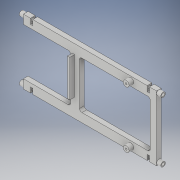
# Autodesk Inventor part: Drivercarrier
Saved by Autodesk Inventor 2019 (Build 230136000, 136)
## iProperties
Created: 2019-01-03
Part Number: Drivercarrier
Material: Generic
Document SubType Name: Modeling
Designer: Martin
Density: 1 g/cm^3
Appearance: Default
Author: Martin
Autodesk Inventor part; units mm, degrees
ref_plane "YZ Plane" through (0, 0, 0) normal (1, 0, 0) x (0, 1, 0)
sketch "Sketch1" plane through (0, 0, 0) normal (0, 0, 1) x (1, 0, 0)
  line L0 (-60, -27.5) -> (60, -27.5)
  line L1 (60, -27.5) -> (60, 27.5)
  line L2 (60, 27.5) -> (-60, 27.5)
  line L3 (-60, 27.5) -> (-60, -27.5)
  line L4 (-60, -27.5) -> (60, 27.5) construction
  line L5 (60, -27.5) -> (-60, 27.5) construction
  point P0 (0, 0)
  dimension "d0" = 120
  dimension "d1" = 55
  constraints: 12 end point, 2 midpoint, 2 parallel, 1 horizontal, 1 perpendicular
  measures "d0" distance of L2.end L1.end
  measures "d1" distance of L1.end L0.end
extrude "Extrusion1" add sketch "Sketch1" against normal blind 4
sketch "Sketch2" plane through (60, -27.5, 0) normal (1, 0, 0) x (0, 0, -1)
  circle A0 centre (2, 2) radius 2
  line L0 (0, 0) -> (4, 0) projected
  line L1 (4, 55) -> (4, 0) projected
  circle A1 centre (2, 2) radius 1.25
  circle A2 centre (2, 53) radius 2
  line L2 (0, 55) -> (4, 55) projected
  circle A3 centre (2, 53) radius 1.25
  line L3 (0, 55) -> (0, 0) projected
  line L4 (0, 55) -> (4, 55)
  line L5 (4, 55) -> (4, 0)
  line L6 (4, 0) -> (0, 0)
  line L7 (0, 0) -> (0, 55)
  point P0 (0, 27.5)
  dimension "d4" = 4
  dimension "d5" = 2.5
  dimension "d6" = 4
  dimension "d7" = 2.5
  constraints: 8 end point, 4 centre point, 4 tangent, 2 coincident, 2 parallel, 1 horizontal, 1 perpendicular
  measures "d4" diameter of A0
  measures "d5" diameter of A1
  measures "d6" diameter of A2
  measures "d7" diameter of A3
extrude "Extrusion2" cut sketch "Sketch2" against normal blind 3.5 contours L1 L0 A0 | A0 L3 A2 L1 | A0 L0 L3 | A2 L2 L1 | L3 L2 A2
extrude "Extrusion3" cut sketch "Sketch2" against normal blind 25 contours A1
extrude "Extrusion4" cut sketch "Sketch2" against normal blind 25 contours A3
sketch "Sketch3" plane through (-60, -27.5, 0) normal (-1, 0, 0) x (0, 0, 1)
  circle A0 centre (-2, 2) radius 2
  circle A1 centre (-2, 53) radius 2
  line L0 (0, 0) -> (-4, 0) projected
  line L1 (-4, 0) -> (-4, 55) projected
  line L2 (0, 55) -> (-4, 55) projected
  line L3 (0, 55) -> (0, 0) projected
  line L4 (-4, 0) -> (0, 0)
  line L5 (0, 0) -> (0, 55)
  line L6 (0, 55) -> (-4, 55)
  line L7 (-4, 55) -> (-4, 0)
  circle A2 centre (-2, 2) radius 1.25 projected
  circle A3 centre (-2, 2) radius 1.25
  circle A4 centre (-2, 53) radius 1.25 projected
  circle A5 centre (-2, 53) radius 1.25
  point P0 (0, 27.5)
  dimension "d14" = 4
  dimension "d15" = 4
  dimension "d16" = 2.5
  dimension "d17" = 2.5
  constraints: 8 end point, 4 centre point, 4 tangent, 2 coincident, 2 parallel, 1 horizontal, 1 perpendicular
  measures "d14" diameter of A0
  measures "d15" diameter of A1
  measures "d16" diameter of A3
  measures "d17" diameter of A5
extrude "Extrusion5" cut sketch "Sketch3" against normal blind 3.5 contours L3 L0 A0 | A0 L1 A1 L3 | A0 L0 L1 | A1 L2 L3 | L1 L2 A1
extrude "Extrusion6" cut sketch "Sketch3" against normal blind 25 contours A4
extrude "Extrusion7" cut sketch "Sketch3" against normal blind 25 contours A2
sketch "Sketch4" plane through (0, 0, 0) normal (0, 0, 1) x (1, 0, 0)
  line L0 (-56.5, 27.5) -> (56.5, 27.5) projected
  line L1 (56.5, -27.5) -> (-56.5, -27.5) projected
  line L2 (-56.5, 27.5) -> (56.5, 27.5)
  line L3 (56.5, 27.5) -> (56.5, -27.5)
  line L4 (56.5, -27.5) -> (-56.5, -27.5)
  line L5 (-56.5, -27.5) -> (-56.5, 27.5)
  line L6 (-73.441, 25.5) -> (75.6749, 25.5) construction
  line L7 (-49.5, 37.9771) -> (-49.5, -42.6684) construction
  line L8 (-50.45, 28) -> (-48.55, 28)
  line L9 (-48.55, 28) -> (-48.55, 23)
  line L10 (-48.55, 23) -> (-50.45, 23)
  line L11 (-50.45, 23) -> (-50.45, 28)
  line L12 (-50.45, 28) -> (-48.55, 23) construction
  line L13 (-48.55, 28) -> (-50.45, 23) construction
  point P0 (0, 0)
  point P1 (-49.5, 25.5)
  dimension "d24" = 2
  dimension "d25" = 7
  dimension "d26" = 1.9
  dimension "d27" = 5
  constraints: 24 end point, 4 parallel, 3 horizontal, 2 midpoint, 2 perpendicular, 2 point on line, 1 vertical
  measures "d24" distance between parallel lines of L0 L6
  measures "d25" distance between parallel lines of L7 L5
  measures "d26" distance of L9.end L10.end
  measures "d27" distance between parallel lines of L10 L8
extrude "Extrusion8" cut sketch "Sketch4" against normal blind 25 contours L11 L8 L9 L0 | L0 L9 L10 L11
ref_plane "Work Plane1" through (0, -27.5, 0) normal (1, 0, 0) x (0, 0, -1)
ref_plane "Work Plane2" through (-48.55, 0, 0) normal (0, 1, 0) x (1, 0, 0)
mirror "Mirror1" about plane through (0, -27.5, 0) normal (1, 0, 0) of "Extrusion8"
mirror "Mirror3" about plane through (-48.55, 0, 0) normal (0, 1, 0) of "Extrusion8", "Mirror1"
sketch "Sketch5" plane through (0, 0, 0) normal (0, 0, 1) x (1, 0, 0)
  line L0 (-20.311, 26.3647) -> (47.689, 26.3647) construction
  line L1 (47.689, 26.3647) -> (47.689, -26.6353) construction
  line L2 (47.689, -26.6353) -> (-20.311, -26.6353) construction
  line L3 (-20.311, -26.6353) -> (-20.311, 26.3647) construction
  line L4 (34.689, 35.6432) -> (34.689, -53.7477) construction
  line L5 (-67.7221, 24) -> (59.2356, 24) construction
  line L6 (-64.2143, -24) -> (60.4803, -24) construction
  line L7 (-93.3625, 0) -> (86.1208, 0) construction
  circle A0 centre (34.689, 24) radius 2.5
  circle A1 centre (34.689, -24) radius 2.5
  line L8 (-15.0696, 19.4646) -> (-13.0566, 19.4646)
  line L9 (-13.0566, 19.4646) -> (-13.0566, -11.8201)
  line L10 (-13.0566, -11.8201) -> (-15.0696, -11.8201)
  line L11 (-15.0696, -11.8201) -> (-15.0696, 19.4646)
  circle A2 centre (34.689, 24) radius 0.75
  circle A3 centre (34.689, -24) radius 0.75
  point P0 (0, 0)
  dimension "d30" = 68
  dimension "d31" = 53
  dimension "d32" = 13
  dimension "d34" = 48
  dimension "d35" = 24
  dimension "d36" = 5
  dimension "d37" = 5
  dimension "d42" = 1.5
  dimension "d43" = 1.5
  constraints: 22 end point, 4 centre point, 4 horizontal, 4 parallel, 4 point on line, 2 coincident, 2 perpendicular, 1 vertical
  measures "d30" distance of L1.end L2.end
  measures "d31" distance of L0.end L1.end
  measures "d32" distance between parallel lines of L1 L4
  measures "d34" distance between parallel lines of L6 L5
  measures "d35" distance between parallel lines of L5 L7
  measures "d36" diameter of A0
  measures "d37" diameter of A1
  measures "d42" diameter of A2
  measures "d43" diameter of A3
extrude "Extrusion9" add sketch "Sketch5" along normal blind 4 contours A0 | A1 | A2 | A3
extrude "Extrusion10" add sketch "Sketch5" along normal blind 4 contours L8 L9 L10 L11
sketch "Sketch6" plane through (34.689, 24, 4) normal (0, 0, 1) x (1, 0, 0)
  circle A0 centre (0, 0) radius 0.75
  circle A1 centre (0, -48.0486) radius 0.75
  point P0 (-34.689, -24)
  dimension "d44" = 1.5
  dimension "d45" = 1.5
  constraints: 2 centre point
  measures "d44" diameter of A0
  measures "d45" diameter of A1
extrude "Extrusion11" cut sketch "Sketch6" against normal blind 7
sketch "Sketch7" plane through (0, 0, 0) normal (0, 0, 1) x (1, 0, 0)
  line L0 (-56.5, -25.5) -> (-56.5, 25.5) projected
  line L1 (-56.5, 20) -> (-16.5, 20)
  line L2 (-16.5, 20) -> (-16.5, -20)
  line L3 (-16.5, -20) -> (-56.5, -20)
  line L4 (-56.5, -20) -> (-56.5, 20)
  line L5 (48.55, 27.5) -> (-48.55, 27.5) projected
  line L6 (-8.902, 20) -> (51.098, 20)
  line L7 (51.098, 20) -> (51.098, -20)
  line L8 (51.098, -20) -> (-8.902, -20)
  line L9 (-8.902, -20) -> (-8.902, 20)
  point P0 (0, 0)
  dimension "d48" = 40
  dimension "d49" = 40
  dimension "d50" = 7.5
  dimension "d51" = 60
  constraints: 16 end point, 4 parallel, 2 horizontal, 2 perpendicular, 1 point on line
  measures "d48" distance of L2.end L3.end
  measures "d49" distance of L1.end L2.end
  measures "d50" distance between parallel lines of L5 L1
  measures "d51" distance of L7.end L8.end
extrude "Extrusion12" cut sketch "Sketch7" against normal blind 7
fillet "Fillet1" radius 2 6 edges at (-16.5, -20, -2) (-16.5, 20, -2) (-8.902, 20, -2) (-8.902, -20, -2) (51.098, 20, -2) (51.098, -20, -2)
body "Solid1"
